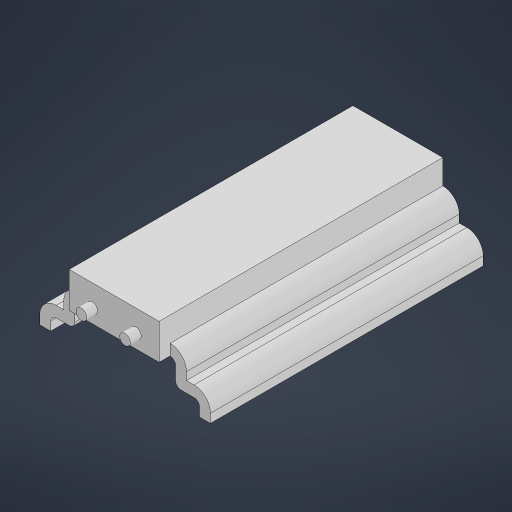
# Autodesk Inventor part: Clamp connector
Saved by Autodesk Inventor 2024 (Build 280153000, 153)
## iProperties
Created: 2024-02-01
Part Number: Clamp connector
Material: Generic
Document SubType Name: Modeling
Designer: chenq
Density: 1 g/cm^3
Appearance: Default
Mass: 198.943 g
Surface Area: 269.925 cm^2
Volume: 198.943 cm^3
Author: chenq
Autodesk Inventor part; units mm, degrees
ref_plane "YZ Plane" through (0, 0, 0) normal (1, 0, 0) x (0, 1, 0)
ref_plane "XZ Plane" through (0, 0, 0) normal (0, 1, 0) x (-1, 0, 0)
ref_plane "XY Plane" through (0, 0, 0) normal (0, 0, 1) x (1, 0, 0)
sketch "Sketch1" plane through (0, 0, 0) normal (0, 1, 0) x (-1, 0, 0)
  line L0 (-23.8125, -82.566) -> (23.8125, -82.566)
  line L1 (23.8125, -82.566) -> (23.8125, 82.566)
  line L2 (23.8125, 82.566) -> (-23.8125, 82.566)
  line L3 (-23.8125, 82.566) -> (-23.8125, -82.566)
  line L4 (-23.8125, -82.566) -> (23.8125, 82.566) construction
  line L5 (23.8125, -82.566) -> (-23.8125, 82.566) construction
  point P0 (0, 0)
  dimension "d0" = 47.625
  dimension "d1" = 165.132
  constraints: 12 end point, 2 midpoint, 2 parallel, 1 horizontal, 1 perpendicular
  measures "d0" distance of L2.end L1.end
  measures "d1" distance of L1.end L0.end
extrude "Extrusion1" add sketch "Sketch1" along normal blind 20.6248
sketch "Sketch5" plane through (-23.8125, 0, -82.566) normal (-1, 0, 0) x (0, 0, 1)
  line L0 (0, 20.6248) -> (165.132, 20.6248) projected
  line L1 (165.132, 0) -> (0, 0) projected
  line L2 (0, 20.6248) -> (165.132, 20.6248)
  line L3 (165.132, 20.6248) -> (165.132, 0)
  line L4 (165.132, 0) -> (0, 0)
  line L5 (0, 0) -> (0, 20.6248)
  point P0 (82.566, 0)
  constraints: 8 end point, 2 parallel, 1 horizontal, 1 perpendicular
extrude "Extrusion4" add sketch "Sketch5" along normal blind 2.3495
sketch "Sketch6" plane through (23.8125, 0, 82.566) normal (1, 0, 0) x (0, 0, -1)
  line L0 (0, 0) -> (0, 20.6248) projected
  line L1 (0, 0) -> (165.132, 0) projected
  line L2 (0, 20.6248) -> (165.132, 20.6248)
  line L3 (165.132, 20.6248) -> (165.132, 0)
  line L4 (165.132, 0) -> (0, 0)
  line L5 (0, 0) -> (0, 20.6248)
  point P0 (82.566, 0)
  constraints: 8 end point, 2 parallel, 1 horizontal, 1 perpendicular
extrude "Extrusion5" add sketch "Sketch6" along normal blind 2.3495
sketch "Sketch7" plane through (-26.162, 0, -82.566) normal (0, 0, -1) x (-1, 0, 0)
  line L0 (0, 0) -> (-52.324, 0) projected
  line L1 (0, -3.175) -> (3.175, -3.175)
  line L2 (0, -3.175) -> (0, 0)
  arc A0 (3.175, -3.175) -> (0, 0) centre (0, -3.175) ccw
  line L3 (-52.324, 0) -> (-52.324, -3.175)
  arc A1 (-52.324, 0) -> (-55.499, -3.175) centre (-52.324, -3.175) ccw
  line L4 (-52.324, -3.175) -> (-55.499, -3.175)
  line L5 (-52.324, 0) -> (-52.324, 6.35)
  line L6 (-52.324, 0) -> (-52.324, 20.6248) projected
  arc A2 (-52.324, 6.35) -> (-61.849, -3.175) centre (-52.324, -3.175) ccw
  line L7 (-55.499, -3.175) -> (-61.849, -3.175)
  line L8 (-55.499, -3.175) -> (-55.499, -10.795)
  line L9 (-55.499, -10.795) -> (-61.849, -10.795)
  line L10 (-61.849, -10.795) -> (-61.849, -3.175)
  line L11 (-55.499, -10.795) -> (-58.674, -10.795)
  arc A3 (-58.674, -13.97) -> (-55.499, -10.795) centre (-58.674, -10.795) ccw
  line L12 (-58.674, -13.97) -> (-66.294, -13.97)
  line L13 (-66.294, -13.97) -> (-66.294, -17.145)
  arc A4 (-66.294, -13.97) -> (-69.469, -17.145) centre (-66.294, -17.145) ccw
  line L14 (-66.294, -17.145) -> (-69.469, -17.145)
  line L15 (-69.469, -17.145) -> (-69.469, -22.225)
  line L16 (-61.849, -13.97) -> (-61.849, -7.62)
  line L17 (-61.849, -7.62) -> (-66.294, -7.62)
  arc A5 (-66.294, -7.62) -> (-75.819, -17.145) centre (-66.294, -17.145) ccw
  line L18 (-69.469, -22.225) -> (-75.819, -22.225)
  line L19 (-75.819, -22.225) -> (-75.819, -17.145)
  line L20 (-69.469, -17.145) -> (-75.819, -17.145)
  line L21 (-26.162, 0) -> (-26.162, 12.6356)
  arc A6 (3.175, -3.175) -> (0, 0) centre (0, -3.175) ccw
  line L22 (0, -3.175) -> (3.175, -3.175)
  arc A7 (9.525, -3.175) -> (0, 6.35) centre (0, -3.175) ccw
  line L23 (3.175, -3.175) -> (9.525, -3.175)
  line L24 (3.175, -3.175) -> (3.175, -10.795)
  line L25 (3.175, -10.795) -> (9.525, -10.795)
  line L26 (9.525, -10.795) -> (9.525, -3.175)
  line L27 (3.175, -10.795) -> (6.35, -10.795)
  arc A8 (3.175, -10.795) -> (6.35, -13.97) centre (6.35, -10.795) ccw
  line L28 (6.35, -13.97) -> (13.97, -13.97)
  line L29 (13.97, -13.97) -> (13.97, -17.145)
  arc A9 (17.145, -17.145) -> (13.97, -13.97) centre (13.97, -17.145) ccw
  line L30 (13.97, -17.145) -> (17.145, -17.145)
  line L31 (17.145, -17.145) -> (17.145, -22.225)
  line L32 (9.525, -13.97) -> (9.525, -7.62)
  line L33 (9.525, -7.62) -> (13.97, -7.62)
  arc A10 (23.495, -17.145) -> (13.97, -7.62) centre (13.97, -17.145) ccw
  line L34 (17.145, -22.225) -> (23.495, -22.225)
  line L35 (23.495, -22.225) -> (23.495, -17.145)
  line L36 (17.145, -17.145) -> (23.495, -17.145)
  line L37 (0, 20.6248) -> (0, 0) projected
  line L38 (0, 0) -> (0, 6.35)
  dimension "d22" = 3.175
  dimension "d23" = 6.35
  dimension "d24" = 7.62
  dimension "d26" = 7.62
  dimension "d29" = 3.175
  dimension "d30" = 5.08
  dimension "d31" = 6.35
  dimension "d32" = 6.35
  constraints: 72 end point, 22 point on circle, 22 symmetric about line, 11 centre point, 9 coincident, 8 horizontal, 5 point on line, 5 vertical, 4 perpendicular, 2 tangent, 1 collinear, 1 midpoint, 5 other
  measures "d22" radius of A0
  measures "d23" distance of L0.end L5.end
  measures "d24" distance of L8.start L8.end
  measures "d26" distance of L12.start L12.end
  measures "d29" distance of L12.end L13.end
  measures "d30" distance of L14.end L15.end
  measures "d31" distance of L16.start L16.end
  measures "d32" distance of L15.end L18.end
extrude "Extrusion6" add sketch "Sketch7" against normal blind 158.75 contours A0 L37 A7 L23 | L23 L26 L25 L24 | L25 L32 L28 A8 | L33 A10 L36 A9 L28 L32 L26 | L35 L34 L31 L36 | A1 L7 A2 L5 | L8 L9 L10 L7 | A3 L12 L16 L9 | L10 L16 L12 A4 L20 A5 L17 | L20 L15 L18 L19
sketch "Sketch8" plane through (-26.162, 0, 82.566) normal (0, 0, 1) x (1, 0, 0)
  line L0 (52.324, 20.6248) -> (0, 20.6248) projected
  line L1 (26.162, 20.6248) -> (26.162, 7.9248)
  line L2 (26.162, 7.9248) -> (38.862, 7.9248)
  line L3 (26.162, 7.9248) -> (13.462, 7.9248)
  circle A0 centre (13.462, 7.9248) radius 3.0687
  circle A1 centre (38.862, 7.9248) radius 3.0687
  point P0 (26.162, 0)
  dimension "d35" = 12.7
  dimension "d36" = 12.7
  dimension "d37" = 12.7
  dimension "d39" = 6.1374
  dimension "d51" = 6.1374
  constraints: 6 end point, 2 centre point, 2 coincident, 1 horizontal, 1 midpoint, 1 perpendicular, 1 vertical
  measures "d35" distance of L1.start L1.end
  measures "d36" distance of L1.end L2.end
  measures "d37" distance of L1.end L3.end
  measures "d39" diameter of A1
  measures "d51" diameter of A0
extrude "Extrusion7" add sketch "Sketch8" along normal blind 6.35
sketch "Sketch9" plane through (26.162, 20.6248, -82.566) normal (0, 0, -1) x (-1, 0, 0)
  line L0 (0, 0) -> (52.324, 0) projected
  line L1 (26.162, 0) -> (26.162, -12.7)
  line L2 (26.162, -12.7) -> (38.862, -12.7)
  line L3 (26.162, -12.7) -> (13.462, -12.7)
  circle A0 centre (13.462, -12.7) radius 3.0687
  circle A1 centre (38.862, -12.7) radius 3.0687
  point P0 (26.162, -20.6248)
  dimension "d42" = 12.7
  dimension "d43" = 12.7
  dimension "d44" = 12.7
  dimension "d49" = 6.1374
  dimension "d50" = 6.1374
  constraints: 6 end point, 2 centre point, 2 coincident, 1 horizontal, 1 midpoint, 1 perpendicular, 1 vertical
  measures "d42" distance of L1.start L1.end
  measures "d43" distance of L1.end L2.end
  measures "d44" distance of L1.end L3.end
  measures "d49" diameter of A0
  measures "d50" diameter of A1
extrude "Extrusion8" add sketch "Sketch9" along normal blind 6.35
body "Solid1"
